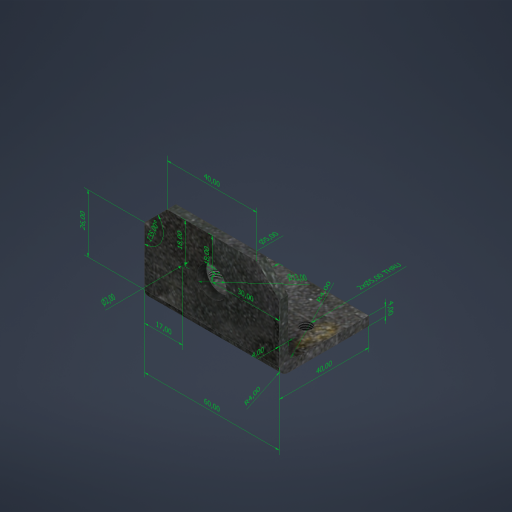
# Autodesk Inventor part: MotorHolder
Saved by Autodesk Inventor 2023 (Build 270158000, 158)
## iProperties
Created: 2022-06-18
Part Number: MotorHolder
Material: Steel
Document SubType Name: Modeling
Designer: Levi
Density: 7.85 g/cm^3
Appearance: Plate
Mass: 134.446 g
Surface Area: 97.3784 cm^2
Volume: 17.1269 cm^3
d13: 60,000 mm
d15: 30,000 mm
d17: 45,00 deg
d20: 4,000 mm
d53: 13,000 mm
d56: 13,000 mm
d57: 2,000 mm
d58: 40,000 mm
d59: 4,000 mm
d60: 0,00 deg
d61: 40,000 mm
d62: 0,00 deg
d63: 10,000 mm
d64: 5,000 mm
d65: 5,000 mm
d76: 4,000 mm
d77: 4,000 mm
Author: Levi
Autodesk Inventor part; units mm, degrees
ref_plane "YZ Plane" through (0, 0, 0) normal (1, 0, 0) x (0, 1, 0)
ref_plane "XZ Plane" through (0, 0, 0) normal (0, 1, 0) x (-1, 0, 0)
ref_plane "XY Plane" through (0, 0, 0) normal (0, 0, 1) x (1, 0, 0)
sketch "Sketch1" plane through (0, 0, 0) normal (0, 0, 1) x (1, 0, 0)
  line L0 (-30.7007, 0.9343) -> (29.2993, 0.9343)
  line L1 (-30.7007, 0.9343) -> (29.2993, 0.9343) construction
  line L2 (29.2993, 0.9343) -> (29.2993, 30.9343)
  line L3 (-30.7007, 30.9343) -> (-30.7007, 0.9343)
  line L4 (-30.7007, 4.9343) -> (29.2993, 4.9343)
  line L5 (-30.7007, 30.9343) -> (-20.7007, 40.9343)
  line L6 (-30.7007, 30.9343) -> (-16.5586, 30.9343) construction
  line L7 (-0.7007, 4.9343) -> (-0.7007, 40.9093) construction
  circle A0 centre (-0.7007, 22.9218) radius 6.5
  line L8 (-0.7007, 22.9218) -> (29.2993, 22.9218) construction
  circle A1 centre (12.2993, 22.9218) radius 1
  line L9 (29.2993, 30.9343) -> (19.2993, 40.9343)
  line L10 (-20.7007, 40.9343) -> (19.2993, 40.9343)
  line L11 (-0.7007, 22.9218) -> (-30.7007, 22.9218) construction
  circle A2 centre (-13.7007, 22.9218) radius 1
  point P0 (-30.2757, 2.8287)
  dimension "d13" = 60
  dimension "d15" = 30
  dimension "d17" = 45
  dimension "d20" = 4
  dimension "d53" = 13
  dimension "d56" = 13
  dimension "d57" = 2
  dimension "d58" = 40
  constraints: 24 end point, 5 perpendicular, 5 point on line, 5 symmetric about line, 4 horizontal, 3 centre point, 3 midpoint, 2 coincident, 2 equal length, 1 other
  measures "d13" distance of L0.start L0.end
  measures "d15" distance of L0.end L2.end
  measures "d17" angle of L6 L5
  measures "d20" distance between parallel lines of L0 L4
  measures "d53" diameter of A0
  measures "d56" distance of point (12.299, 22.922) L8.start
  measures "d57" diameter of A1
  measures "d58" distance of L5.end L9.end
extrude "Extrusion3" add sketch "Sketch1" against normal blind 4 contours L3 L5 L10 L9 L2 L4
extrude "Extrusion4" add sketch "Sketch1" against normal blind 40 contours L3 L4 L2 L0
sketch "Sketch4" plane through (-30.7007, 4.9343, -4) normal (0, 1, 0) x (1, 0, 0)
  line L0 (60, 0) -> (60, 36) projected
  line L1 (60, 18) -> (0, 18) construction
  line L2 (0, 0) -> (0, 36) projected
  line L3 (0, 36) -> (60, 36) projected
  line L4 (30, 36) -> (30, 0) construction
  line L5 (10, 0) -> (50, 0) projected
  circle A0 centre (50, 18) radius 2.5
  circle A1 centre (10, 18) radius 2.5
  point P0 (30.7007, -4)
  dimension "d63" = 10
  dimension "d64" = 5
  constraints: 4 end point, 4 midpoint, 2 centre point, 1 point on line, 1 symmetric about line, 1 other
  measures "d63" distance from line of L0 A0.centre
  measures "d64" diameter of A0
hole "Hole3" at (19.2993, 4.9343, -22) at (-20.7007, 4.9343, -22) direction (0, -1, 0) diameter 5 end through all
thread "Thread1" size "M6x1" class "6H" standard "ANSI Metric M Profile" full length
thread "Thread2" size "M6x1" class "6H" standard "ANSI Metric M Profile" full length
fillet "Fillet2" radius 4 1 edges at (-0.7007, 4.9343, -4)
fillet "Fillet3" radius 4 1 edges at (-0.7007, 0.9343, 0)
body "Solid2"
